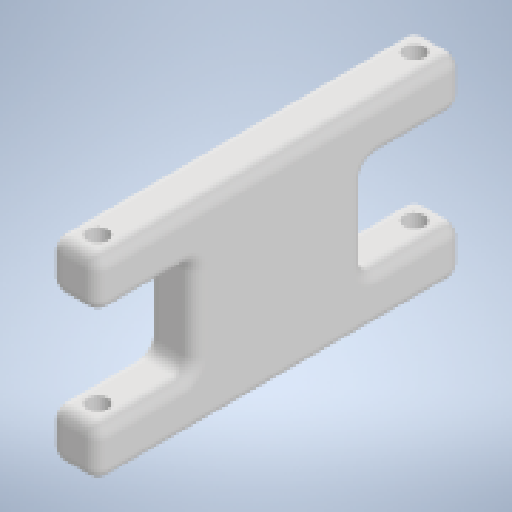
# Autodesk Inventor part: swing pusher
Saved by Autodesk Inventor 2023 (Build 270158000, 158)
## iProperties
Created: 2023-01-25
Part Number: swing pusher
Material: Generic
Document SubType Name: Modeling
Designer: Gabriel - T3 CAD
Density: 1 g/cm^3
Appearance: Default
Mass: 40.324 g
Surface Area: 106.324 cm^2
Volume: 40.324 cm^3
Author: Gabriel - T3 CAD
Autodesk Inventor part; units mm, degrees
ref_plane "YZ Plane" through (0, 0, 0) normal (1, 0, 0) x (0, 1, 0)
ref_plane "XZ Plane" through (0, 0, 0) normal (0, 1, 0) x (-1, 0, 0)
ref_plane "XY Plane" through (0, 0, 0) normal (0, 0, 1) x (1, 0, 0)
sketch "Sketch1" plane through (0, 0, 0) normal (0, 1, 0) x (-1, 0, 0)
  line L0 (0, 0) -> (12.7, 0)
  line L1 (12.7, 0) -> (12.7, 95.25)
  line L2 (12.7, 95.25) -> (0, 95.25)
  line L3 (0, 95.25) -> (0, 0)
  circle A0 centre (6.35, 6.35) radius 2.5797
  circle A1 centre (6.35, 88.9) radius 2.5797
  dimension "d0" = 12.7
  dimension "d1" = 95.25
  dimension "d2" = 6.35
  dimension "d3" = 6.35
  dimension "d4" = 5.1594
  dimension "d5" = 6.35
  dimension "d6" = 5.1594
  dimension "d7" = 6.35
  constraints: 8 end point, 2 centre point, 2 parallel, 1 horizontal, 1 perpendicular
  measures "d0" distance of L2.end L1.end
  measures "d1" distance of L1.end L0.end
  measures "d2" distance from line of L0 A0.centre
  measures "d3" distance from line of L1 A0.centre
  measures "d4" diameter of A0
  measures "d5" distance from line of L1 A1.centre
  measures "d6" diameter of A1
  measures "d7" distance from line of L2 A1.centre
extrude "Extrusion1" add sketch "Sketch1" along normal blind 50.8
sketch "Sketch3" plane through (0, 0, 95.25) normal (1, 0, 0) x (0, 0, -1)
  line L0 (95.25, 0) -> (95.25, 50.8) projected
  line L1 (95.25, 38.1) -> (69.85, 38.1)
  line L2 (95.25, 38.1) -> (120.65, 38.1) construction
  line L3 (69.85, 38.1) -> (69.85, 12.7)
  line L4 (69.85, 12.7) -> (95.25, 12.7)
  line L5 (0, 50.8) -> (95.25, 50.8) projected
  line L6 (95.25, 50.8) -> (0, 50.8) projected
  line L7 (69.85, 50.8) -> (69.85, 38.1)
  line L8 (69.85, 12.7) -> (69.85, 0)
  line L9 (95.25, 0) -> (0, 0) projected
  line L10 (0, 0) -> (0, 50.8) projected
  line L11 (0, 38.1) -> (25.4, 38.1)
  line L12 (25.4, 38.1) -> (25.4, 12.7)
  line L13 (25.4, 12.7) -> (0, 12.7)
  line L14 (0, 12.7) -> (0, 38.1)
  dimension "d24" = 25.4
  dimension "d25" = 180
  dimension "d26" = 25.4
  dimension "d27" = 12.7
  dimension "d31" = 25.4
  dimension "d32" = 25.4
  constraints: 20 end point, 6 point on line, 4 perpendicular, 3 collinear, 2 horizontal, 2 parallel
  measures "d24" distance of L1.start L1.end
  measures "d25" angle of L1 L2
  measures "d26" distance of L1.end L3.end
  measures "d27" distance between parallel lines of L5 L1
  measures "d31" distance of L12.end L13.end
  measures "d32" distance of L11.end L12.end
extrude "Extrusion3" cut sketch "Sketch3" against normal through all contours L4 L3 L1 L0 | L10 L11 L12 L13
fillet "Fillet2" radius 3.175 36 edges at (0, 50.8, 47.625) (-6.35, 50.8, 95.25) (-6.35, 0, 0) (-12.7, 50.8, 47.625) (0, 0, 47.625) (-12.7, 0, 47.625) (-6.35, 38.1, 25.4) (0, 25.4, 25.4) (0, 38.1, 12.7) (-12.7, 38.1, 12.7) (-12.7, 6.35, 0) (0, 6.35, 0) (-6.35, 38.1, 0) (-12.7, 44.45, 0) (0, 44.45, 0) (-6.35, 50.8, 0) (-12.7, 25.4, 25.4) (-6.35, 0, 95.25) (0, 6.35, 95.25) (-12.7, 6.35, 95.25) (0, 12.7, 82.55) (-12.7, 12.7, 82.55) (-6.35, 12.7, 95.25) (-6.35, 38.1, 69.85) (0, 38.1, 82.55) (-12.7, 38.1, 82.55) (-6.35, 38.1, 95.25) (0, 44.45, 95.25) (-12.7, 44.45, 95.25) (-6.35, 12.7, 0) (0, 12.7, 12.7) (-12.7, 12.7, 12.7) (-6.35, 12.7, 25.4) (-6.35, 12.7, 69.85) (0, 25.4, 69.85) (-12.7, 25.4, 69.85)
equation "\"d31\" = d24"
body "Solid1"
